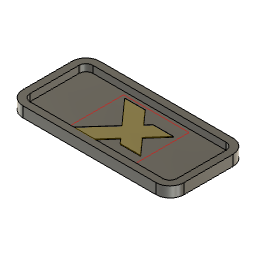
GIX_Desk_Tray (Autodesk Fusion 360 design; units mm, degrees)
Autodesk Fusion 360 part; units mm, degrees
box "BoxPrimitive1" add length 139.7 width 292.1 height 19.05 placed x (0, 1, 0) y (-1, 0, 0) z (0, 0, 1) at (292.1, 0, 0)
fillet "Fillet1" radius 25.4 4 edges at (0, 0, 9.525) (0, 139.7, 9.525) (292.1, 0, 9.525) (292.1, 139.7, 9.525)
sketch "Sketch2" plane through (0, 0, 19.05) normal (0, 0, 1) x (-1, 0, 0)
  arc A0 (-292.1, -114.3) -> (-266.7, -139.7) centre (-266.7, -114.3) ccw
  line L0 (-266.7, -139.7) -> (-25.4, -139.7)
  arc A1 (-25.4, -139.7) -> (0, -114.3) centre (-25.4, -114.3) ccw
  line L1 (0, -114.3) -> (0, -25.4)
  arc A2 (0, -25.4) -> (-25.4, 0) centre (-25.4, -25.4) ccw
  line L2 (-25.4, 0) -> (-266.7, 0)
  arc A3 (-266.7, 0) -> (-292.1, -25.4) centre (-266.7, -25.4) ccw
  line L3 (-292.1, -25.4) -> (-292.1, -114.3)
  line L4 (-12.7, -114.3) -> (-12.7, -25.4)
  arc A4 (-12.7, -25.4) -> (-25.4, -12.7) centre (-25.4, -25.4) ccw
  line L5 (-25.4, -12.7) -> (-266.7, -12.7)
  arc A5 (-266.7, -12.7) -> (-279.4, -25.4) centre (-266.7, -25.4) ccw
  line L6 (-279.4, -25.4) -> (-279.4, -114.3)
  arc A6 (-279.4, -114.3) -> (-266.7, -127) centre (-266.7, -114.3) ccw
  line L7 (-266.7, -127) -> (-25.4, -127)
  arc A7 (-25.4, -127) -> (-12.7, -114.3) centre (-25.4, -114.3) ccw
  point P0 (-292.1, 0)
  point P1 (0, -139.7)
  constraint tangent A6 L7
  constraint tangent L7 A7
  constraint tangent L5 A5
  constraint tangent L4 A7
  constraint tangent A5 L6
  constraint tangent L6 A6
  constraint tangent A4 L5
  constraint tangent L4 A4
extrude "Extrude1" cut sketch "Sketch2" against normal blind 12.7 contours L4 A4 L5 A5 L6 A6 L7 A7
sketch "Sketch3" plane through (0, 0, 6.35) normal (0, 0, 1) x (-1, 0, 0)
  arc A0 (-25.4, -127) -> (-12.7, -114.3) centre (-25.4, -114.3) ccw
  line L0 (-12.7, -114.3) -> (-12.7, -25.4)
  arc A1 (-12.7, -25.4) -> (-25.4, -12.7) centre (-25.4, -25.4) ccw
  line L1 (-25.4, -12.7) -> (-266.7, -12.7)
  arc A2 (-266.7, -12.7) -> (-279.4, -25.4) centre (-266.7, -25.4) ccw
  line L2 (-279.4, -25.4) -> (-279.4, -114.3)
  arc A3 (-279.4, -114.3) -> (-266.7, -127) centre (-266.7, -114.3) ccw
  line L3 (-266.7, -127) -> (-25.4, -127)
  line L4 (-94.1365, -115.8394) -> (-131.1548, -115.8394)
  line L5 (-161.648, -99.7247) -> (-198.5274, -99.7247)
  line L6 (-161.6096, -40.1639) -> (-198.5361, -40.1639)
  line L7 (-93.4326, -23.8572) -> (-130.9835, -23.8572)
  line L8 (-93.4326, -23.8572) -> (-134.9646, -70.048)
  line L9 (-153.5362, -90.703) -> (-161.648, -99.7247)
  line L10 (-161.6096, -40.1639) -> (-153.5494, -49.2039)
  line L11 (-134.9646, -70.048) -> (-94.1365, -115.8394)
  line L12 (-130.9835, -23.8572) -> (-153.5494, -49.2039)
  line L13 (-172.017, -69.9473) -> (-198.5274, -99.7247)
  line L14 (-131.1548, -115.8394) -> (-153.5362, -90.703)
  line L15 (-172.017, -69.9473) -> (-198.5361, -40.1639)
  constraint horizontal L4
  constraint parallel L3 L5
  constraint parallel L3 L6
  constraint horizontal L7
  constraint coincident L8.end L10
  constraint collinear L8 L9
  constraint collinear L10 L11
  constraint coincident L13.start L14
  constraint collinear L12 L13
  constraint collinear L14 L15
extrude "Extrude2" add sketch "Sketch3" along normal blind 1.27 contours L4 L5 L6 L7 L8 L9 L10 L11 L12 L13 L14 L15
